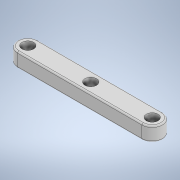
# Autodesk Inventor part: G-1
Saved by Autodesk Inventor 2021 (Build 250183000, 183)
## iProperties
Created: 2021-06-26
Part Number: G-1
Material: Generic
Document SubType Name: Modeling
Designer: Ranjita
Density: 1 g/cm^3
Appearance: Default
Author: Ranjita
Autodesk Inventor part; units mm, degrees
ref_plane "YZ Plane" through (0, 0, 0) normal (1, 0, 0) x (0, 1, 0)
ref_plane "XZ Plane" through (0, 0, 0) normal (0, 1, 0) x (-1, 0, 0)
ref_plane "XY Plane" through (0, 0, 0) normal (0, 0, 1) x (1, 0, 0)
sketch "Sketch1" plane through (0, 0, 0) normal (0, 1, 0) x (-1, 0, 0)
  line L0 (0, 0) -> (28.33, 0) construction
  line L1 (0, -2.33) -> (28.33, -2.33)
  line L2 (28.33, 2.33) -> (0, 2.33)
  arc A0 (0, 2.33) -> (0, -2.33) centre (0, 0) ccw
  arc A1 (28.33, -2.33) -> (28.33, 2.33) centre (28.33, 0) ccw
  circle A2 centre (28.33, 0) radius 1.33
  circle A3 centre (0, 0) radius 1.33
  circle A4 centre (14, 0) radius 1.33
  point P0 (14.165, 0)
  dimension "d0" = 28.33
  dimension "d1" = 4.66
  dimension "d2" = 2.66
  dimension "d3" = 14
  constraints: 8 end point, 5 centre point, 4 point on circle, 4 tangent, 2 coincident, 2 equal radius, 1 horizontal, 1 midpoint, 1 parallel, 1 point on line
  measures "d0" distance of L1.start L1.end
  measures "d1" distance between parallel lines of L2 L1
  measures "d2" diameter of A3
  measures "d3" distance of A3.centre A4.centre
extrude "Extrusion1" add sketch "Sketch1" along normal blind 3.33
fillet "Fillet1" radius 0.33 8 edges at (2.33, 3.33, 0) (-14.165, 3.33, -2.33) (-30.66, 3.33, 0) (-14.165, 3.33, 2.33) (2.33, 0, 0) (-14.165, 0, -2.33) (-30.66, 0, 0) (-14.165, 0, 2.33)
body "Solid1"
